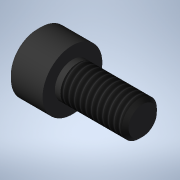
# Autodesk Inventor part: SCB5-10
Saved by Autodesk Inventor 2021 (Build 250183000, 183)
## iProperties
Created: 2025-07-10
Part Number: SCB5-10
Material: Generic
Catalog Web Link: www.cadenas.de
Description: SCB-Hexagon Socket Head Cap Screws - Stainless Steel
Vendor: MISUMI
Document SubType Name: Modeling
Designer: psAdmin
Manufacturer: MISUMI
Mass: 0.438216 g
Surface Area: 4.26199 cm^2
Volume: 0.438216 cm^3
Density: 1 g/cm^3
Appearance: PSOLRGB-175-175-175
Category: PARTsolutions
Company: MISUMI
Title: SCB5-10
Author: Cadenas PARTsolutions
Comments: Hexagon Socket Head Cap Screws - Stainless Steel
PSOL_IDENT_0: {$CADENAS_DATA/23d-libs/misumi/metric/27_screws_nuts/scb_fa.prj},153 {VTYP=3D},{NB=SCB5-10},{LINA=SC
PSOL_IDENT_1: B5-10},{NN=SCB},{DATE=03.06.2021 03:35:43},{GEOMDATE=23.02.2012 00:00:00},{VERSION=},{LINEID=40},{WB
PSOL_IDENT_2: VAR=L},{WBNUMERIC=L}  {NB=SCB5-10},{LINA=SCB5-10},{KT=DUMMY},{PN=SCB5-10},{MAT=SUSXM7(30430 Stainles
PSOL_IDENT_3: s Steel)},{SC=A2-70},{M=5},{L=10},{LL=Full Thread},{L1=22},{TYPE=SCB},{M1=5.0},{L0=6,8,10,12,14,15,1
PSOL_IDENT_4: 6,18,20,22,25,30,35,40,45,50},{MP=5x0.8},{P=0.8},{A=8.5},{E=5.0},{B=4.0},{V=0.50}
NB: SCB5-10
NN: SCB
NT: Hexagon Socket Head Cap Screws - Stainless Steel
NBSYN: $PN.
LINA: SCB5-10
CATALOG: Misumi
PN: SCB5-10
MAT: 302HQ Stainless Steel
SC: A2-70
M: 5
L: 10
LL: Full Thread
MP: 5x0.8
A: 8.5
E: 5
B: 4
SUPPLIER: MISUMI
ARTICLENO: SCB5-10
BOMINFO: SCB5-10
CREATOR: CADENAS GmbH
Autodesk Inventor part; units mm, degrees
sketch "Sketch_1" plane through (0, 0, 0) normal (0, 0, 1) x (1, 0, 0)
  line L0 (10, 0) -> (-5, 0)
  line L1 (-5, 0) -> (-5, 3.75)
  line L2 (-5, 3.75) -> (-4.5, 4.25)
  line L3 (-4.5, 4.25) -> (0, 4.25)
  line L4 (0, 4.25) -> (0, 2.5)
  line L5 (0, 2.5) -> (9.5095, 2.5)
  line L6 (9.5095, 2.5) -> (10, 2.0095)
  line L7 (10, 2.0095) -> (10, 0)
  line L8 (10, 0) -> (-5, 0)
  constraints: 18 end point
revolve "Revolution1" add sketch "Sketch_1" angle 360 about axis through (10, 0, 0) along (1, 0, 0)
thread "Thread1" size "M5x0.8" class "6g" standard "ISO Metric profile" length 8.7095
sketch "Sketch2" plane through (-5, 0, 0) normal (-1, 0, 0) x (0, 0, 1)
  point P0 (0, 0)
hole "Hole1" at (-5, 0, 0) direction (1, 0, 0) diameter 4 depth 2.5 tip angle 150
sketch "Sketch_3" plane through (-5, 0, 0) normal (1, 0, 0) x (0, 0, -1)
  line L0 (-2, -1.1547) -> (0, -2.3094)
  line L1 (0, -2.3094) -> (2, -1.1547)
  line L2 (2, -1.1547) -> (2, 1.1547)
  line L3 (2, 1.1547) -> (0, 2.3094)
  line L4 (0, 2.3094) -> (-2, 1.1547)
  line L5 (-2, 1.1547) -> (-2, -1.1547)
  constraints: 12 end point
extrude "Extrusion1" cut sketch "Sketch_3" along normal blind 2.5
ref_plane "bolt_XY" through (0, 0, 0) normal (1, 0, 0) x (0, 0, -1)
ref_plane "bolt_YZ" through (0, 0, 0) normal (0, 0, -1) x (0, 1, 0)
ref_plane "bolt_ZX" through (0, 0, 0) normal (0, 1, 0) x (1, 0, 0)
ref_plane "nut_XY" through (10, 0, 0) normal (1, 0, 0) x (0, 0, -1)
ref_plane "nut_YZ" through (10, 0, 0) normal (0, 0, -1) x (0, 1, 0)
ref_plane "nut_ZX" through (10, 0, 0) normal (0, 1, 0) x (1, 0, 0)
body "Solid1"
